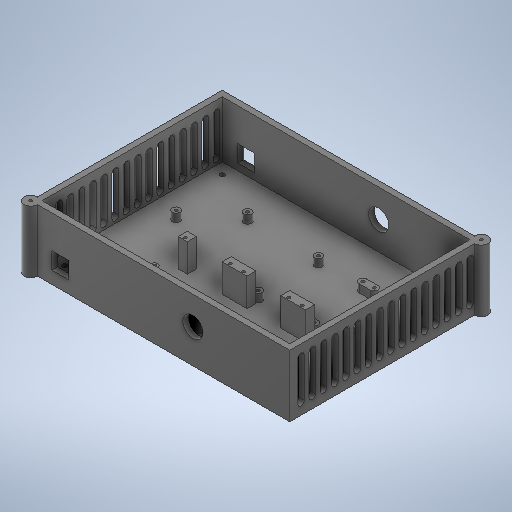
# Autodesk Inventor part: Power Box (24V)
Saved by Autodesk Inventor 2026.2 (Build 302298010, 298A)
## iProperties
Created: 2026-05-01
Part Number: Power Box (24V)
Material: ABS Plastic
Document SubType Name: Modeling
Designer: chanh
Density: 1.06 g/cm^3
Appearance: Smooth - White
Author: chanh
Autodesk Inventor part; units mm, degrees
ref_plane "YZ Plane" through (0, 0, 0) normal (1, 0, 0) x (0, 1, 0)
ref_plane "XZ Plane" through (0, 0, 0) normal (0, 1, 0) x (-1, 0, 0)
ref_plane "XY Plane" through (0, 0, 0) normal (0, 0, 1) x (1, 0, 0)
sketch "Sketch1" plane through (0, 0, 0) normal (0, 1, 0) x (-1, 0, 0)
  line L0 (115, 85) -> (-115, 85)
  line L1 (-115, 85) -> (-115, -85)
  line L2 (-115, -85) -> (115, -85)
  line L3 (115, -85) -> (115, 85)
  line L4 (115, 85) -> (-115, -85) construction
  line L5 (-115, 85) -> (115, -85) construction
  point P0 (0, 0)
  dimension "d0" = 230
  dimension "d1" = 170
  constraints: 12 end point, 2 midpoint, 2 parallel, 1 horizontal, 1 perpendicular
  measures "d0" distance of L1.end L2.end
  measures "d1" distance of L0.end L1.end
extrude "Extrusion1" add sketch "Sketch1" along normal blind 55
shell "Shell1" thickness 5 removed faces 1 at (38.3333, 55, -28.3333)
sketch "Sketch2" plane through (-110, 5, -80) normal (0, 1, 0) x (1, 0, 0)
  line L0 (171, -100) -> (211, -100) construction
  line L1 (211, -100) -> (211, -140) construction
  line L2 (211, -140) -> (171, -140) construction
  line L3 (171, -140) -> (171, -100) construction
  line L4 (171, -100) -> (211, -140) construction
  line L5 (211, -100) -> (171, -140) construction
  line L6 (119, -100) -> (159, -100) construction
  line L7 (159, -100) -> (159, -140) construction
  line L8 (159, -140) -> (119, -140) construction
  line L9 (119, -140) -> (119, -100) construction
  line L10 (119, -100) -> (159, -140) construction
  line L11 (159, -100) -> (119, -140) construction
  line L12 (67, -100) -> (107, -100) construction
  line L13 (107, -100) -> (107, -140) construction
  line L14 (107, -140) -> (67, -140) construction
  line L15 (67, -140) -> (67, -100) construction
  line L16 (67, -100) -> (107, -140) construction
  line L17 (107, -100) -> (67, -140) construction
  line L18 (220, -160) -> (220, 0) construction
  line L19 (220, 0) -> (0, 0) construction
  line L20 (0, 0) -> (0, -160) construction
  line L21 (0, -160) -> (220, -160) construction
  line L22 (6, -130.8) -> (59.3, -130.8) construction
  line L23 (59.3, -130.8) -> (59.3, -29.2) construction
  line L24 (59.3, -29.2) -> (6, -29.2) construction
  line L25 (6, -29.2) -> (6, -130.8) construction
  line L26 (6, -130.8) -> (59.3, -29.2) construction
  line L27 (59.3, -130.8) -> (6, -29.2) construction
  line L28 (211, -36.5) -> (171.5, -36.5) construction
  line L29 (171.5, -36.5) -> (171.5, -90) construction
  line L30 (171.5, -90) -> (211, -90) construction
  line L31 (211, -90) -> (211, -36.5) construction
  line L32 (211, -36.5) -> (171.5, -90) construction
  line L33 (171.5, -36.5) -> (211, -90) construction
  line L34 (161.5, -36.5) -> (122, -36.5) construction
  line L35 (122, -36.5) -> (122, -90) construction
  line L36 (122, -90) -> (161.5, -90) construction
  line L37 (161.5, -90) -> (161.5, -36.5) construction
  line L38 (161.5, -36.5) -> (122, -90) construction
  line L39 (122, -36.5) -> (161.5, -90) construction
  point P0 (110, -80)
  point P1 (191, -120)
  point P2 (139, -120)
  point P3 (87, -120)
  point P4 (32.65, -80)
  point P5 (0, -80)
  point P6 (56.8, -116.83)
  point P7 (56.8, -34.28)
  point P8 (23.8, -64.73)
  point P9 (191.25, -63.25)
  point P10 (141.75, -63.25)
  dimension "d5" = 40
  dimension "d6" = 40
  dimension "d7" = 40
  dimension "d8" = 12
  dimension "d9" = 12
  dimension "d10" = 9
  dimension "d11" = 20
  dimension "d12" = 101.6
  dimension "d13" = 53.3
  dimension "d14" = 6
  dimension "d15" = 2.5
  dimension "d16" = 13.97
  dimension "d17" = 96.52
  dimension "d18" = 33
  dimension "d19" = 52.1
  dimension "d20" = 53.5
  dimension "d21" = 39.5
  dimension "d22" = 53.5
  dimension "d23" = 39.5
  dimension "d24" = 9
  dimension "d25" = 10
  dimension "d26" = 10
  constraints: 72 end point, 13 midpoint, 12 parallel, 9 perpendicular, 6 horizontal, 4 horizontal alignment, 1 vertical alignment
  measures "d5" distance of L0.start L0.end
  measures "d6" distance of L6.start L6.end
  measures "d7" distance of L12.start L12.end
  measures "d8" distance between parallel lines of L3 L7
  measures "d9" distance between parallel lines of L9 L13
  measures "d10" distance between parallel lines of L18 L1
  measures "d11" distance between parallel lines of L2 L21
  measures "d12" distance of L24.end L22.start
  measures "d13" distance of L23.end L24.end
  measures "d14" distance between parallel lines of L20 L25
  measures "d15" distance from line of L23 point (56.8, -34.28)
  measures "d16" distance from line of L22 point (56.8, -116.83)
  measures "d17" distance from line of point (56.8, -34.28) L22
  measures "d18" horizontal distance of point (23.8, -64.73) point (56.8, -116.83)
  measures "d19" vertical distance of point (23.8, -64.73) point (56.8, -116.83)
  measures "d20" distance of L30.end L28.start
  measures "d21" distance of L29.end L30.end
  measures "d22" distance of L37.start L34.start
  measures "d23" distance of L35.end L37.start
  measures "d24" distance between parallel lines of L18 L31
  measures "d25" distance between parallel lines of L29 L37
  measures "d26" distance between parallel lines of L0 L30
sketch "Sketch3" plane through (-110, 5, -80) normal (0, 1, 0) x (1, 0, 0)
  circle A0 centre (23.8, -64.73) radius 3.5
  circle A1 centre (56.8, -34.28) radius 3.5
  circle A2 centre (56.8, -116.83) radius 3
  circle A3 centre (122, -36.5) radius 3.5
  circle A4 centre (122, -90) radius 3.5
  circle A5 centre (161.5, -90) radius 3.5
  circle A6 centre (161.5, -36.5) radius 3.5
  circle A7 centre (171.5, -36.5) radius 3.5
  circle A8 centre (171.5, -90) radius 3.5
  circle A9 centre (211, -90) radius 3.5
  circle A10 centre (211, -36.5) radius 3.5
  line L0 (161.5, -33) -> (171.5, -33)
  line L1 (161.5, -40) -> (171.5, -40)
  line L2 (161.5, -86.5) -> (171.5, -86.5)
  line L3 (171.5, -93.5) -> (161.5, -93.5)
  point P0 (110, -80)
  dimension "d27" = 7
  dimension "d28" = 7
  dimension "d38" = 6
  constraints: 11 centre point, 11 coincident, 8 end point, 8 equal radius, 8 point on circle, 4 tangent, 1 parallel
  measures "d27" diameter of A0
  measures "d28" diameter of A3
  measures "d38" diameter of A2
extrude "Extrusion2" add sketch "Sketch3" along normal blind 7
sketch "Sketch4" plane through (-86.2, 12, -15.27) normal (0, 1, 0) x (1, 0, 0)
  circle A0 centre (33, 30.45) radius 3.5 projected
  line L0 (137.7, 31.73) -> (147.7, 31.73) projected
  arc A1 (147.7, 24.73) -> (147.7, 31.73) centre (147.7, 28.23) ccw projected
  line L1 (147.7, 24.73) -> (137.7, 24.73) projected
  arc A2 (137.7, 31.73) -> (137.7, 24.73) centre (137.7, 28.23) ccw projected
  circle A3 centre (187.2, 28.23) radius 3.5 projected
  circle A4 centre (98.2, 28.23) radius 3.5 projected
  circle A5 centre (33, -52.1) radius 3 projected
  line L2 (137.7, -21.77) -> (147.7, -21.77) projected
  arc A6 (147.7, -28.77) -> (147.7, -21.77) centre (147.7, -25.27) ccw projected
  line L3 (147.7, -28.77) -> (137.7, -28.77) projected
  arc A7 (137.7, -21.77) -> (137.7, -28.77) centre (137.7, -25.27) ccw projected
  circle A8 centre (187.2, -25.27) radius 3.5 projected
  circle A9 centre (98.2, -25.27) radius 3.5 projected
  circle A10 centre (0, 0) radius 3.5 projected
  line L4 (196.2, -95.27) -> (196.2, 64.73) projected
  line L5 (196.2, 64.73) -> (-23.8, 64.73) projected
  line L6 (-23.8, 64.73) -> (-23.8, -95.27) projected
  line L7 (-23.8, -95.27) -> (196.2, -95.27) projected
  point P0 (86.2, -15.27)
hole "Hole1" at (-86.2, 12, -15.27) at (-53.2, 12, -45.72) at (-53.2, 12, 36.83) at (12, 12, 10) at (12, 12, -43.5) at (51.5, 12, -43.5) at (61.5, 12, -43.5) at (101, 12, -43.5) at (51.5, 12, 10) at (61.5, 12, 10) at (101, 12, 10) direction (0, -1, 0) diameter 2.7 depth 7
sketch "Sketch5" plane through (-110, 5, -80) normal (0, 1, 0) x (1, 0, 0)
  circle A0 centre (67, -140) radius 4
  circle A1 centre (107, -140) radius 4
  circle A2 centre (119, -140) radius 4
  circle A3 centre (159, -140) radius 4
  circle A4 centre (171, -140) radius 4
  circle A5 centre (211, -140) radius 4
  line L0 (107, -136) -> (119, -136)
  line L1 (119, -136) -> (119, -144)
  line L2 (119, -144) -> (107, -144)
  line L3 (107, -144) -> (107, -136)
  line L4 (159, -136) -> (171, -136)
  line L5 (171, -136) -> (171, -144)
  line L6 (171, -144) -> (159, -144)
  line L7 (159, -144) -> (159, -136)
  line L8 (102, -94) -> (124, -94)
  line L9 (124, -94) -> (124, -102)
  line L10 (124, -102) -> (102, -102)
  line L11 (102, -102) -> (102, -94)
  line L12 (107, -100) -> (119, -100) construction
  line L13 (154, -94) -> (176, -94)
  line L14 (176, -94) -> (176, -102)
  line L15 (176, -102) -> (154, -102)
  line L16 (154, -102) -> (154, -94)
  line L17 (159, -100) -> (171, -100) construction
  line L18 (63, -94) -> (71, -94)
  line L19 (71, -94) -> (71, -102)
  line L20 (71, -102) -> (63, -102)
  line L21 (63, -102) -> (63, -94)
  line L22 (207, -94) -> (215, -94)
  line L23 (215, -94) -> (215, -102)
  line L24 (215, -102) -> (207, -102)
  line L25 (207, -102) -> (207, -94)
  point P0 (110, -80)
  point P1 (67, -100)
  point P2 (211, -100)
  point P3 (113, -100)
  point P4 (113, -102)
  point P5 (165, -102)
  point P6 (165, -100)
  point P7 (67, -102)
  point P8 (211, -102)
  point P9 (107, -144)
  dimension "d39" = 8
  dimension "d40" = 2
  dimension "d41" = 8
  dimension "d42" = 22
  dimension "d43" = 2
  dimension "d44" = 8
  dimension "d45" = 22
  dimension "d46" = 8
  dimension "d47" = 8
  dimension "d48" = 8
  dimension "d49" = 8
  dimension "d50" = 2
  dimension "d51" = 2
  constraints: 52 end point, 12 parallel, 8 horizontal, 7 coincident, 6 midpoint, 6 perpendicular, 6 vertical alignment, 2 centre point, 2 point on line, 1 equal radius, 16 other
  measures "d39" diameter of A0
  measures "d40" distance from line of L10 L12.start
  measures "d41" distance between parallel lines of L8 L10
  measures "d42" distance between parallel lines of L9 L11
  measures "d43" distance from line of L15 L17.start
  measures "d44" distance between parallel lines of L13 L15
  measures "d45" distance between parallel lines of L14 L16
  measures "d46" distance of L20.end L18.start
  measures "d47" distance between parallel lines of L19 L21
  measures "d48" distance of L24.end L25.end
  measures "d49" distance between parallel lines of L23 L25
  measures "d50" distance from line of L20 point (67, -100)
  measures "d51" distance from line of L24 point (211, -100)
extrude "Extrusion3" add sketch "Sketch5" along normal blind 25
sketch "Sketch6" plane through (-110, 30, -80) normal (0, 1, 0) x (1, 0, 0)
  point P0 (110, -80)
  point P1 (67, -100)
  point P2 (107, -100)
  point P3 (119, -100)
  point P4 (159, -100)
  point P5 (171, -100)
  point P6 (211, -100)
  point P7 (67, -140)
  point P8 (107, -140)
  point P9 (119, -140)
  point P10 (159, -140)
  point P11 (171, -140)
  point P12 (211, -140)
hole "Hole2" at (-43, 30, 20) at (-3, 30, 20) at (9, 30, 20) at (49, 30, 20) at (61, 30, 20) at (101, 30, 20) at (101, 30, 60) at (61, 30, 60) at (49, 30, 60) at (9, 30, 60) at (-3, 30, 60) at (-43, 30, 60) direction (0, -1, 0) diameter 2.7 depth 7
sketch "Sketch7" plane through (-110, 5, -80) normal (0, 1, 0) x (1, 0, 0)
  line L0 (220, -160) -> (0, -160) projected
  line L1 (0, -160) -> (0, 0) projected
  line L2 (0, 0) -> (220, 0) projected
  line L3 (220, 0) -> (220, -160) projected
  line L4 (225, -165) -> (225, 5) projected
  line L5 (225, 5) -> (-5, 5) projected
  line L6 (-5, 5) -> (-5, -165) projected
  line L7 (-5, -165) -> (225, -165) projected
  line L8 (110, 0) -> (110, -160) construction
  line L9 (220, -80) -> (0, -80) construction
  point P0 (110, -80)
  point P1 (10, -10)
  point P2 (210, -10)
  point P3 (10, -150)
  point P4 (210, -150)
  dimension "d61" = 10
  dimension "d62" = 10
  constraints: 4 end point, 4 midpoint, 3 symmetric about line
  measures "d61" distance from line of L2 point (10, -10)
  measures "d62" distance from line of L1 point (10, -10)
hole "Hole3" at (-100, 5, -70) at (100, 5, -70) at (-100, 5, 70) at (100, 5, 70) direction (0, -1, 0) diameter 4.2 end through all
sketch "Sketch8" plane through (-110, 5, -80) normal (1, 0, 0) x (0, 0, -1)
  line L0 (-152, 40) -> (-152, 5)
  line L1 (-158, 5) -> (-158, 40)
  arc A0 (-152, 40) -> (-158, 40) centre (-155, 40) ccw
  arc A1 (-158, 5) -> (-152, 5) centre (-155, 5) ccw
  line L2 (5, -5) -> (-165, -5) projected
  line L3 (-165, -5) -> (-165, 50) projected
  line L4 (5, 50) -> (-165, 50) projected
  line L5 (5, -5) -> (5, 50) projected
  line L6 (-155, 40) -> (-155, 5) construction
  point P0 (-80, -5)
  point P1 (-155, 22.5)
  point P2 (-165, 22.5)
  dimension "d70" = 35
  dimension "d71" = 6
  dimension "d72" = 10
  constraints: 6 end point, 4 point on circle, 4 tangent, 2 centre point, 2 midpoint, 1 horizontal alignment, 1 parallel, 1 vertical
  measures "d70" distance of L6.start L6.end
  measures "d71" distance between parallel lines of L0 L1
  measures "d72" distance between parallel lines of L3 L6
extrude "Extrusion4" cut sketch "Sketch8" against normal through all contours L0 A1 L1 A0
pattern_linear "Rectangular Pattern1" count 16 spacing 10 along (0, 0, -1) of "Extrusion4"
mirror "Mirror1" about plane through (0, 0, 0) normal (1, 0, 0) of "Extrusion4", "Rectangular Pattern1"
sketch "Sketch9" plane through (-115, 0, 85) normal (0, 0, 1) x (1, 0, 0)
  line L0 (32.3, 12) -> (25.3, 12) projected
  line L1 (18.8, 26) -> (33.8, 26)
  line L2 (33.8, 26) -> (33.8, 11)
  line L3 (33.8, 11) -> (18.8, 11)
  line L4 (18.8, 11) -> (18.8, 26)
  line L5 (64.8, 12) -> (58.8, 12) projected
  line L6 (129, 5) -> (129, 30) projected
  line L7 (129, 5) -> (129, 30) projected
  line L8 (159, 5) -> (159, 30) projected
  line L9 (129, 30) -> (159, 30) construction
  circle A0 centre (144, 30) radius 9
  point P0 (115, 0)
  dimension "d78" = 15
  dimension "d79" = 15
  dimension "d81" = 14
  dimension "d82" = 46
  dimension "d83" = 18
  constraints: 10 end point, 2 horizontal, 2 parallel, 1 centre point, 1 midpoint, 1 perpendicular
  measures "d78" distance of L2.end L3.end
  measures "d79" distance of L1.end L2.end
  measures "d81" distance between parallel lines of L1 L0
  measures "d82" distance from line of L4 L5.start
  measures "d83" diameter of A0
extrude "Extrusion5" cut sketch "Sketch9" against normal blind 10
sketch "Sketch10" plane through (115, 0, -85) normal (0, 0, -1) x (-1, 0, 0)
  circle A0 centre (86, 30) radius 9 projected
  line L0 (211.2, 26) -> (211.2, 11) projected
  line L1 (196.2, 26) -> (211.2, 26) projected
  line L2 (196.2, 11) -> (196.2, 26) projected
  line L3 (211.2, 11) -> (196.2, 11) projected
  point P0 (115, 0)
extrude "Extrusion6" cut sketch "Sketch10" against normal up to surface (5 mm away)
sketch "Sketch11" plane through (0, 55, 0) normal (0, 1, 0) x (1, 0, 0)
  line L0 (110, -80) -> (-110, -80) projected
  line L1 (-110, -80) -> (-110, 80) projected
  line L2 (-110, 80) -> (110, 80) projected
  line L3 (110, 80) -> (110, -80) projected
  line L4 (115, -85) -> (115, 85) projected
  line L5 (115, 85) -> (-115, 85) projected
  line L6 (-115, 85) -> (-115, -85) projected
  line L7 (-115, -85) -> (115, -85) projected
  circle A0 centre (115, 85) radius 6
  circle A1 centre (-115, -85) radius 6
  point P0 (0, 0)
  point P1 (-115, -79)
  point P2 (-109, -85)
  dimension "d88" = 12
  constraints: 2 centre point, 2 coincident, 1 equal radius
  measures "d88" diameter of A1
extrude "Extrusion7" add sketch "Sketch11" against normal up to surface (55 mm away) contours A0 L5 L4 | L4 L5 A0 | A1 L6 L7 picked at (-118.8848, -84.1854)
sketch "Sketch12" plane through (0, 55, 0) normal (0, 1, 0) x (1, 0, 0)
  line L0 (109, 85) -> (-115, 85) projected
  line L1 (-115, 85) -> (-115, -79) projected
  arc A0 (-115, -79) -> (-109, -85) centre (-115, -85) ccw projected
  line L2 (-109, -85) -> (115, -85) projected
  line L3 (115, -85) -> (115, 79) projected
  arc A1 (115, 79) -> (109, 85) centre (115, 85) ccw projected
  line L4 (110, -80) -> (-110, -80) projected
  line L5 (-110, -80) -> (-110, 80) projected
  line L6 (-110, 80) -> (110, 80) projected
  line L7 (110, 80) -> (110, -80) projected
  point P0 (0, 0)
hole "Hole4" at (-115, 55, 85) at (115, 55, -85) direction (0, -1, 0) diameter 2.7 depth 7
equation "\"d9\" = d8"
body "Solid1"
